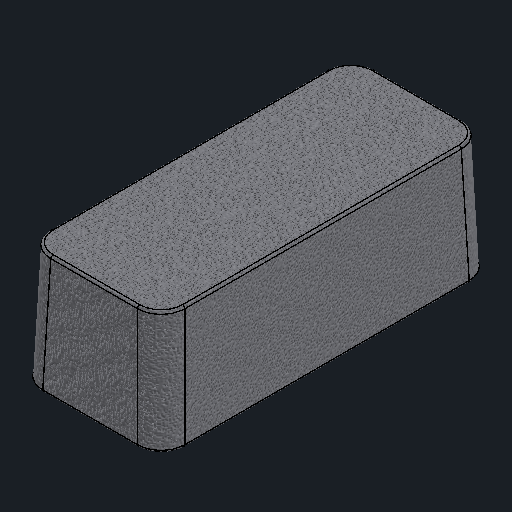
# Autodesk Inventor part: Drive
Saved by Autodesk Inventor 2026.2 (Build 302298000, 298)
## iProperties
Created: 2026-05-18
Part Number: Drive
Material: Steel, Cast
Document SubType Name: Modeling
Designer: JoshuaEah
Density: 7.85 g/cm^3
Appearance: Iron - Cast
Author: JoshuaEah
Autodesk Inventor part; units mm, degrees
ref_plane "YZ Plane" through (0, 0, 0) normal (1, 0, 0) x (0, 1, 0)
ref_plane "XZ Plane" through (0, 0, 0) normal (0, 1, 0) x (-1, 0, 0)
ref_plane "XY Plane" through (0, 0, 0) normal (0, 0, 1) x (1, 0, 0)
sketch "Sketch1" plane through (0, 0, 0) normal (0, 1, 0) x (-1, 0, 0)
  line L0 (0, 0) -> (-38.1, 0)
  line L1 (-38.1, 0) -> (-38.1, -88.9)
  line L2 (-38.1, -88.9) -> (0, -88.9)
  line L3 (0, -88.9) -> (0, 0)
  dimension "d0" = 38.1
  dimension "d1" = 88.9
  constraints: 8 end point, 2 parallel, 1 coincident, 1 horizontal, 1 perpendicular
  measures "d0" distance of L2.end L1.end
  measures "d1" distance of L1.end L0.end
extrude "Extrusion1" add sketch "Sketch1" along normal blind 31.75 draft -2
fillet "Fillet1" radius 6.35 4 edges at (0.5544, 15.875, -0.5544) (37.5456, 15.875, -88.3456) (0.5544, 15.875, -88.3456) (37.5456, 15.875, -0.5544)
fillet "Fillet2" radius 0.635 16 edges at (35.133, 31.75, -2.967) (19.05, 31.75, -1.1087) (2.967, 31.75, -2.967) (1.1087, 31.75, -44.45) (2.967, 31.75, -85.933) (19.05, 31.75, -87.7913) (35.133, 31.75, -85.933) (36.9913, 31.75, -44.45) (36.2417, 0, -87.0417) (19.05, 0, -88.9) (1.8583, 0, -87.0417) (0, 0, -44.45) (1.8583, 0, -1.8583) (19.05, 0, 0) (36.2417, 0, -1.8583) (38.1, 0, -44.45)
body "Solid1"
